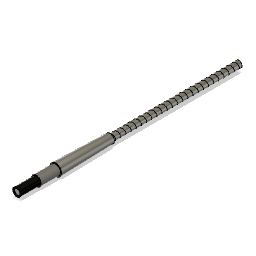
Spektrometer Rotrics Adapter - Top - Well Adapter V2 (Autodesk Fusion 360 archive; units mm, degrees)
design "OceanOnsight Spektrometer"
Autodesk Fusion 360 part; units mm, degrees
sketch "Skizze1" plane through (0, 0, 0) normal (0, 0, 1) x (1, 0, 0)
  circle A0 centre (0, 0) radius 3.25
  dimension "d46" = 6.5
  constraint coincident A0.centre origin
  measures "d46" diameter of A0
extrude "Extrusion1" add sketch "Skizze1" along normal blind 15
sketch "Skizze2" plane through (0, 0, 0) normal (0, 0, -1) x (-1, 0, 0)
  circle A0 centre (0, 0) radius 3.25
  circle A1 centre (0, 0) radius 3.75
  dimension "d49" = 7.5
  constraint coincident A0.centre A1.centre
  measures "d49" diameter of A1
extrude "Extrusion2" add sketch "Skizze2" along normal blind 15 contours A0 | A1
sketch "Skizze3" plane through (0, 0, 15) normal (0, 0, 1) x (1, 0, 0)
  circle A0 centre (0, 0) radius 3.25
  circle A1 centre (0, 0) radius 2.25
  dimension "d52" = 4.5
  constraint coincident A0.centre A1.centre
  measures "d52" diameter of A1
extrude "Extrusion3" cut sketch "Skizze3" against normal blind 0.5 contours A1
sketch "Skizze4" plane through (0, 0, -15) normal (0, 0, -1) x (-1, 0, 0)
  circle A0 centre (0, 0) radius 3.75
  circle A1 centre (0, 0) radius 4.5
  dimension "d55" = 9
  constraint concentric A0 A1
  measures "d55" diameter of A1
ref_plane "Arbeitsebene1" through (0, 0, -57) normal (0, 0, -1) x (-1, 0, 0)
sketch "Skizze5" plane through (0, 0, -57) normal (0, 0, -1) x (1, 0, 0)
  circle A0 centre (0, 0) radius 3.5
  dimension "d57" = 7
  constraint coincident A0.centre origin
  measures "d57" diameter of A0
loft "Erhebung1" add profiles "Skizze4", "Skizze5" section 1 contours A0 | A1 section 2
sketch "Skizze6" plane through (0, 0, -57) normal (0, 0, -1) x (-1, 0, 0)
  circle A0 centre (0, 0) radius 3.5
  circle A1 centre (0, 0) radius 2.5
  dimension "d58" = 5
  constraint coincident A0.centre A1.centre
  measures "d58" diameter of A1
extrude "Extrusion4" add sketch "Skizze6" along normal blind 100 contours A1
coil "Grundkörper Spirale1" cut diameter 5 section circle size 0.25 inside turns 25 pitch 4 right hand placed x (-1, 0, 0) y (0, -1, 0) z (0, 0, 1) at (0, 0, -157)
